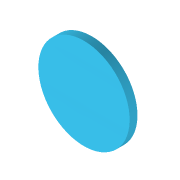
# Autodesk Inventor part: 50_ETL_Membrane_Mould_Lower_v0
Saved by Autodesk Inventor 2022 (Build 260153000, 153)
## iProperties
Created: 2021-12-31
Part Number: 50_ETL_Membrane_Mould_Lower_v0
Material: Generisch
Document SubType Name: Modeling
Designer: diederichbenedict
Density: 1 g/cm^3
Appearance: Türkis
Author: diederichbenedict
Autodesk Inventor part; units mm, degrees
ref_plane "YZ Plane" through (0, 0, 0) normal (1, 0, 0) x (0, 1, 0)
ref_plane "XZ Plane" through (0, 0, 0) normal (0, 1, 0) x (-1, 0, 0)
ref_plane "XY Plane" through (0, 0, 0) normal (0, 0, 1) x (1, 0, 0)
sketch "Skizze1" plane through (0, 0, 0) normal (1, 0, 0) x (0, 1, 0)
  line L0 (0, 0) -> (0, -0.6)
  line L1 (-25, 0) -> (0, 0) projected
  line L2 (-25, -0.6) -> (0, -0.6) projected
  line L3 (-20.8023, -2.2) -> (-4.1977, -2.2) projected
  line L4 (-20.6011, -1.9989) -> (-21.4, -1.2)
  line L5 (-21.4, -1.2) -> (-21.4, 0)
  line L6 (-25, 0) -> (-25, -0.6)
  line L7 (-22.8485, -0.6) -> (-20.8497, -2.5989)
  line L8 (-21.0508, -2.8) -> (-3.9492, -2.8) projected
  line L9 (0, -0.6) -> (5, -0.6)
  line L10 (5, -0.6) -> (5, 2.4)
  line L11 (-12.5, -6.6891) -> (-12.5, -2.8)
  line L12 (0, 4.2178) -> (0, -8.5069) projected
  line L13 (5, 2.4) -> (-12.5, 2.4)
  line L14 (-19.2569, -1) -> (-5.7431, -1) projected
  line L15 (-18.5, -0.8) -> (-6.5, -0.8) construction
  line L16 (-6.5, -0.8) -> (-6.5, -1) construction
  line L17 (-6.5, -1) -> (-18.5, -1) construction
  line L18 (-18.5, -1) -> (-18.5, -0.8) construction
  line L19 (-18.5, -0.8) -> (-12.5, -0.9) construction
  line L20 (-6.5, -0.8) -> (-18.5, -1) construction
  line L21 (-12.5, 2.4) -> (-12.5, -0.8)
  line L22 (-12.5, -0.8) -> (-6.4, -0.7983) construction
  line L23 (-6.4, -0.7983) -> (-6.4, -1) construction
  line L24 (-12.5, -0.8) -> (-6.4, -0.7983) construction
  line L25 (-6.4, -0.7983) -> (-6.4, -1) construction
  line L26 (-12.5, -0.8) -> (-6.4, -0.7983)
  line L27 (-6.4, -0.7983) -> (-6.4, -1)
  line L28 (-6.5, -1) -> (-6.5167, -1)
  line L29 (-5.7431, -1) -> (-6.1949, -1.0051)
  line L30 (-3.6, 0) -> (0, 0)
  line L31 (-5.9715, -1.2285) -> (-6.1949, -1.0051)
  line L32 (-5, -2.2) -> (-4.4683, -2.2)
  line L33 (-5, -2.2) -> (-5.3167, -2.2)
  line L34 (-5.3167, -2.2) -> (-3.6196, -2.2) construction
  line L35 (-3.2, -1.2) -> (-3.2, 0)
  line L36 (-4.1989, -2.1989) -> (-3.2, -1.2)
  line L37 (-20.8023, -2.2) -> (-4.1977, -2.2) projected
  line L38 (-4.1977, -2.2) -> (-4.9977, -2.2)
  line L39 (-5.7431, -1) -> (-4.5431, -2.2)
  point P0 (-2.1515, -0.6)
  point P1 (-22.8485, -0.6)
  point P2 (-12.5, -1)
  point P3 (-12.5, -0.6)
  point P4 (-21.4, -0.6)
  point P5 (-12.5, 0)
  dimension "d0" = 5
  dimension "d1" = 3
  dimension "d2" = 17.1016
  dimension "d3" = 8.5508
  dimension "d4" = 12
  dimension "d5" = 0.2
  dimension "d6" = 6.1
  constraints: 64 end point, 5 horizontal, 5 midpoint, 5 point on line, 4 perpendicular, 4 vertical, 3 parallel, 20 other
  measures "d0" distance of L0.end L9.end
  measures "d1" distance of L9.end L10.end
  measures "d2" distance of L7.end L8.end
  measures "d3" distance from line of L11 L8.end
  measures "d4" distance of L16.end L17.end
  measures "d5" distance of L16.end L15.end
  measures "d6" distance of L21.end L22.end
revolve "Umdrehung1" add sketch "Skizze1" angle 360 about axis through (0, -12.5, 2.4) along (0, 0, -1) contours L12 L13 L10 L9 L0 | L1 L21 L13 L12 | L35 L2 L21 L1 | L35 L36 L3 L39 L14 L27 L26 L21 L2
equation "\"d3\" = 0.5 * d2"
